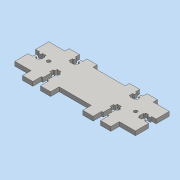
# Autodesk Inventor part: X-Anchor_Top
Saved by Autodesk Inventor 2016 SP1 (Build 200210100, 210)
## iProperties
Created: 2016-01-20
Part Number: X-Anchor_Top
Material: Generic
Document SubType Name: Modeling
Designer: Mohamed A.
Density: 1 g/cm^3
Appearance: Default
Author: Mohamed A.
Autodesk Inventor part; units mm, degrees
ref_plane "YZ Plane" through (0, 0, 0) normal (1, 0, 0) x (0, 1, 0)
ref_plane "XZ Plane" through (0, 0, 0) normal (0, 1, 0) x (-1, 0, 0)
ref_plane "XY Plane" through (0, 0, 0) normal (0, 0, 1) x (1, 0, 0)
sketch "Sketch3" plane through (0, 0, 0) normal (0, 0, 1) x (1, 0, 0)
  line L0 (-42.7335, 16.5) -> (42.7335, 16.5)
  line L1 (42.7335, 16.5) -> (42.7335, -16.5)
  line L2 (42.7335, -16.5) -> (-42.7335, -16.5)
  line L3 (-42.7335, -16.5) -> (-42.7335, 16.5)
  line L4 (-42.7335, 16.5) -> (42.7335, -16.5) construction
  line L5 (42.7335, 16.5) -> (-42.7335, -16.5) construction
  point P0 (0, 0)
  dimension "d5" = 33
  dimension "d6" = 85.467
  constraints: 12 end point, 2 midpoint, 2 parallel, 1 horizontal, 1 perpendicular
  measures "d5" distance of L0.end L1.end
  measures "d6" distance between parallel lines of L3 L1
extrude "Extrusion2" add sketch "Sketch3" along normal blind 3
sketch "Sketch4" plane through (0, 0, 3) normal (0, 0, 1) x (1, 0, 0)
  line L0 (-42.7335, 16.5) -> (-42.7335, -16.5) projected
  line L1 (42.7335, -16.5) -> (42.7335, 16.5) projected
  line L2 (-42.7335, -16.5) -> (42.7335, -16.5) projected
  line L3 (42.7335, -16.5) -> (31.2905, -16.5)
  line L4 (31.2905, -16.5) -> (31.2905, -10.5)
  line L5 (31.2905, -10.5) -> (42.7335, -10.5)
  line L6 (42.7335, -10.5) -> (42.7335, -16.5)
  line L7 (21.3575, -16.5) -> (21.3575, 22.3854) construction
  line L8 (22.8575, -16.5) -> (19.8575, -16.5)
  line L9 (19.8575, -16.5) -> (19.8575, -0.5)
  line L10 (19.8575, -0.5) -> (22.8575, -0.5)
  line L11 (22.8575, -0.5) -> (22.8575, -16.5)
  line L12 (18.7075, -2.1) -> (24.0075, -2.1)
  line L13 (24.0075, -2.1) -> (24.0075, -4.5)
  line L14 (24.0075, -4.5) -> (18.7075, -4.5)
  line L15 (18.7075, -4.5) -> (18.7075, -2.1)
  line L16 (0, 33.54) -> (0, -25.8799) construction
  line L17 (-42.7335, -16.5) -> (-31.2905, -16.5)
  line L18 (-31.2905, -16.5) -> (-31.2905, -10.5)
  line L19 (-31.2905, -10.5) -> (-42.7335, -10.5)
  line L20 (-42.7335, -10.5) -> (-42.7335, -16.5)
  line L21 (-22.8575, -16.5) -> (-19.8575, -16.5)
  line L22 (-19.8575, -16.5) -> (-19.8575, -0.5)
  line L23 (-19.8575, -0.5) -> (-22.8575, -0.5)
  line L24 (-22.8575, -0.5) -> (-22.8575, -16.5)
  line L25 (-18.7075, -2.1) -> (-24.0075, -2.1)
  line L26 (-24.0075, -2.1) -> (-24.0075, -4.5)
  line L27 (-24.0075, -4.5) -> (-18.7075, -4.5)
  line L28 (-18.7075, -4.5) -> (-18.7075, -2.1)
  line L29 (11.4245, -16.5) -> (-11.4245, -16.5)
  line L30 (-11.4245, -16.5) -> (-11.4245, -10.5)
  line L31 (-11.4245, -10.5) -> (11.4245, -10.5)
  line L32 (11.4245, -10.5) -> (11.4245, -16.5)
  line L33 (58.2331, 0) -> (-60.3586, 0) construction
  line L34 (42.7335, 16.5) -> (31.2905, 16.5)
  line L35 (31.2905, 16.5) -> (31.2905, 13.5)
  line L36 (31.2905, 13.5) -> (42.7335, 13.5)
  line L37 (42.7335, 13.5) -> (42.7335, 16.5)
  line L38 (42.7335, 16.5) -> (-42.7335, 16.5) projected
  line L39 (11.4245, 16.5) -> (-11.4245, 16.5)
  line L40 (-11.4245, 16.5) -> (-11.4245, 13.5)
  line L41 (-11.4245, 13.5) -> (11.4245, 13.5)
  line L42 (11.4245, 13.5) -> (11.4245, 16.5)
  line L43 (-42.7335, 16.5) -> (-31.2905, 16.5)
  line L44 (-31.2905, 16.5) -> (-31.2905, 13.5)
  line L45 (-31.2905, 13.5) -> (-42.7335, 13.5)
  line L46 (-42.7335, 13.5) -> (-42.7335, 16.5)
  line L47 (22.8575, 16.5) -> (19.8575, 16.5)
  line L48 (19.8575, 16.5) -> (19.8575, 8.5)
  line L49 (19.8575, 8.5) -> (22.8575, 8.5)
  line L50 (22.8575, 8.5) -> (22.8575, 16.5)
  line L51 (18.7075, 9.1) -> (24.0075, 9.1)
  line L52 (24.0075, 9.1) -> (24.0075, 11.5)
  line L53 (24.0075, 11.5) -> (18.7075, 11.5)
  line L54 (18.7075, 11.5) -> (18.7075, 9.1)
  line L55 (-22.8575, 16.5) -> (-19.8575, 16.5)
  line L56 (-19.8575, 16.5) -> (-19.8575, 8.5)
  line L57 (-19.8575, 8.5) -> (-22.8575, 8.5)
  line L58 (-22.8575, 8.5) -> (-22.8575, 16.5)
  line L59 (-18.7075, 9.1) -> (-24.0075, 9.1)
  line L60 (-24.0075, 9.1) -> (-24.0075, 11.5)
  line L61 (-24.0075, 11.5) -> (-18.7075, 11.5)
  line L62 (-18.7075, 11.5) -> (-18.7075, 9.1)
  line L63 (42.7335, 1.5) -> (32.1415, 1.5) construction
  line L64 (42.7335, 3) -> (34.7335, 3)
  line L65 (34.7335, 3) -> (34.7335, 0)
  line L66 (34.7335, 0) -> (42.7335, 0)
  line L67 (42.7335, 0) -> (42.7335, 3)
  line L68 (35.3335, 4.15) -> (37.7335, 4.15)
  line L69 (37.7335, 4.15) -> (37.7335, -1.15)
  line L70 (37.7335, -1.15) -> (35.3335, -1.15)
  line L71 (35.3335, -1.15) -> (35.3335, 4.15)
  line L72 (24.0075, -16.5) -> (18.7075, -16.5)
  line L73 (18.7075, -16.5) -> (18.7075, -10.5)
  line L74 (18.7075, -10.5) -> (24.0075, -10.5)
  line L75 (24.0075, -10.5) -> (24.0075, -16.5)
  line L76 (-18.7075, -16.5) -> (-24.0075, -16.5)
  line L77 (-24.0075, -16.5) -> (-24.0075, -10.5)
  line L78 (-24.0075, -10.5) -> (-18.7075, -10.5)
  line L79 (-18.7075, -10.5) -> (-18.7075, -16.5)
  line L80 (24.0075, 16.5) -> (18.7075, 16.5)
  line L81 (18.7075, 16.5) -> (18.7075, 13.5)
  line L82 (18.7075, 13.5) -> (24.0075, 13.5)
  line L83 (24.0075, 13.5) -> (24.0075, 16.5)
  line L84 (-18.7075, 16.5) -> (-24.0075, 16.5)
  line L85 (-24.0075, 16.5) -> (-24.0075, 13.5)
  line L86 (-24.0075, 13.5) -> (-18.7075, 13.5)
  line L87 (-18.7075, 13.5) -> (-18.7075, 16.5)
  line L88 (42.7335, 4.15) -> (39.7335, 4.15)
  line L89 (39.7335, 4.15) -> (39.7335, -1.15)
  line L90 (39.7335, -1.15) -> (42.7335, -1.15)
  line L91 (42.7335, -1.15) -> (42.7335, 4.15)
  line L92 (-42.7335, 3) -> (-34.7335, 3)
  line L93 (-34.7335, 3) -> (-34.7335, 0)
  line L94 (-34.7335, 0) -> (-42.7335, 0)
  line L95 (-42.7335, 0) -> (-42.7335, 3)
  line L96 (-35.3335, 4.15) -> (-37.7335, 4.15)
  line L97 (-37.7335, 4.15) -> (-37.7335, -1.15)
  line L98 (-37.7335, -1.15) -> (-35.3335, -1.15)
  line L99 (-35.3335, -1.15) -> (-35.3335, 4.15)
  line L100 (-42.7335, 4.15) -> (-39.7335, 4.15)
  line L101 (-39.7335, 4.15) -> (-39.7335, -1.15)
  line L102 (-39.7335, -1.15) -> (-42.7335, -1.15)
  line L103 (-42.7335, -1.15) -> (-42.7335, 4.15)
  circle A0 centre (-30.8335, 1.5) radius 1.25
  circle A1 centre (30.8335, 1.5) radius 1.25
  dimension "d12" = 11.443
  dimension "d13" = 6
  dimension "d17" = 3
  dimension "d18" = 16
  dimension "d20" = 5.3
  dimension "d21" = 2.4
  dimension "d22" = 6
  dimension "d27" = 3
  dimension "d28" = 8
  dimension "d29" = 5
  dimension "d30" = 8
  dimension "d31" = 3
  dimension "d32" = 2.4
  dimension "d33" = 5.3
  dimension "d34" = 5
  dimension "d35" = 3
  dimension "d38" = 2.5
  dimension "d39" = 11.9
  dimension "d40" = 24
  dimension "d41" = 12
  dimension "d42" = 2.5
  dimension "d43" = 11.9
  dimension "d44" = 12
  dimension "d45" = 7.283
  dimension "d46" = 7.283
  dimension "d47" = 7.283
  dimension "d48" = 7.283
  constraints: 200 end point, 32 parallel, 31 symmetric about line, 19 collinear, 19 horizontal, 16 perpendicular, 15 point on line, 4 equal length, 3 vertical, 2 centre point, 5 other
  measures "d12" distance of L4.end L5.end
  measures "d13" distance of L3.end L4.end
  measures "d17" distance of L9.end L10.end
  measures "d18" distance of L8.end L9.end
  measures "d20" distance of L13.end L14.end
  measures "d21" distance of L12.end L13.end
  measures "d22" distance between parallel lines of L14 L5
  measures "d27" distance of L35.end L34.end
  measures "d28" distance of L48.end L47.end
  measures "d29" distance between parallel lines of L38 L53
  measures "d30" distance of L66.end L65.end
  measures "d31" distance of L65.end L64.end
  measures "d32" distance of L69.end L70.end
  measures "d33" distance of L68.end L69.end
  measures "d34" distance between parallel lines of L67 L69
  measures "d35" distance between parallel lines of L91 L89
  measures "d38" diameter of A0
  measures "d39" distance from line of A0.centre L0
  measures "d40" distance between parallel lines of L19 L45
  measures "d41" distance from line of L45 A0.centre
  measures "d42" diameter of A1
  measures "d43" distance from line of L1 A1.centre
  measures "d44" distance from line of A1.centre L36
  measures "d45" distance between parallel lines of L4 L75
  measures "d46" distance between parallel lines of L32 L73
  measures "d47" distance between parallel lines of L30 L79
  measures "d48" distance between parallel lines of L18 L77
extrude "Extrusion3" cut sketch "Sketch4" against normal up to next contours L38 L44 L45 L0 | L100 L101 L92 L0 | L38 L58 L86 L85 | L92 L101 L94 L0 | L38 L56 L86 L58 | L94 L101 L102 L0 | L92 L97 L94 L101 | L38 L87 L86 L56 | L86 L56 L61 L58 | L97 L96 L99 L92 | L92 L99 L94 L97 | L61 L56 L59 L58 | L58 L59 L60 L61 | L19 L18 L2 L0 | L94 L99 L98 L97 | L92 L93 L94 L99 | L38 L42 L41 L40 | L61 L62 L59 L56 | L59 L56 L57 L58 | L38 L48 L82 L81 | L77 L78 L24 L2 | L38 L50 L82 L48 | L24 L78 L22 L2 | L38 L83 L82 L50 | L82 L50 L53 L48 | L22 L78 L79 L2 | L24 L27 L22 L78 | L53 L50 L51 L48 | L48 L51 L54 L53 | L27 L26 L25 L24 | L24 L25 L22 L27 | L34 L1 L36 L35 | L53 L52 L51 L50 | L51 L50 L49 L48 | L30 L31 L32 L2 | L22 L25 L28 L27 | L24 L23 L22 L25 | L73 L74 L9 L2 | L1 L64 L89 L88 | L9 L74 L11 L2 | L1 L66 L89 L64 | L11 L74 L75 L2 | L9 L14 L11 L74 | L1 L90 L89 L66 | L89 L66 L69 L64 | L14 L15 L12 L9 | L9 L12 L11 L14 | L69 L66 L71 L64 | L64 L71 L68 L69 | L4 L5 L1 L2 | L11 L12 L13 L14 | L9 L10 L11 L12 | L69 L70 L71 L66 | L71 L66 L65 L64 | A0 | A1
equation "\"d41\" = 0.5 * d40"
equation "\"d44\" = d41"
equation "\"d46\" = d45"
equation "\"d47\" = d46"
body "Solid2"
